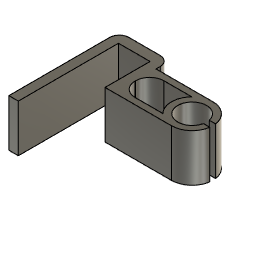
auto-top-off-clip (Autodesk Fusion 360 design; units mm, degrees)
Autodesk Fusion 360 part; units mm, degrees
note: some values were not read from the file. Set by a fixed rule: which sketch regions a step uses.
sketch "Sketch1" plane through (0, 0, 0) normal (0, 0, 1) x (1, 0, 0)
  line L0 (0, 0) -> (0, 31.75)
  line L1 (0, 31.75) -> (10, 31.75)
  line L2 (10, 31.75) -> (10, 15.875)
  line L3 (10, 15.875) -> (12, 15.875)
  line L4 (0, 0) -> (-3, 0)
  line L5 (-3, 0) -> (-3, 35)
  line L6 (-3, 35) -> (13, 35)
  line L7 (13, 35) -> (13, 17.5)
  line L8 (13, 17.5) -> (10, 17.5)
  circle A0 centre (31.0292, 24.0805) radius 4.572
  circle A1 centre (31.0292, 24.0805) radius 6.572
  line L9 (13, 17.5) -> (31.0468, 17.5)
  line L10 (31.0468, 17.5) -> (31.0468, 19.5)
  line L11 (31.0468, 19.5) -> (13, 19.5)
  line L12 (13, 19.5) -> (13, 17.5)
  line L13 (31.0292, 28.6525) -> (12.2404, 28.6525)
  line L14 (12.2404, 28.6525) -> (12.2404, 30.6525)
  line L15 (12.2404, 30.6525) -> (31.0292, 30.6525)
  line L16 (31.0292, 30.6525) -> (31.0292, 28.6525)
  line L17 (38, 25) -> (24.0584, 25)
  line L18 (24.0584, 25) -> (24.0584, 23.1611)
  line L19 (24.0584, 23.1611) -> (38, 23.1611)
  line L20 (38, 23.1611) -> (38, 25)
  line L21 (38, 25) -> (24.0584, 23.1611) construction
  line L22 (24.0584, 25) -> (38, 23.1611) construction
  point P0 (31.0292, 24.0805)
  dimension "d1" = 31.75
  dimension "d2" = 10
  dimension "d3" = 15.875
  dimension "d4" = 2
  dimension "d5" = 9.144
  dimension "d6" = 2
  dimension "d11" = 2
  dimension "d12" = 2
  constraint coincident L0.start L4.start
  constraint vertical L0
  constraint perpendicular L0 L1
  constraint perpendicular L1 L2
  constraint perpendicular L2 L3
  constraint perpendicular L0 L4
  constraint perpendicular L4 L5
  constraint perpendicular L5 L6
  constraint perpendicular L4 L7
  constraint coincident L2 L8.end
  constraint perpendicular L2 L8
  constraint horizontal L9
  constraint vertical L10
  constraint horizontal L11
  constraint vertical L12
  constraint horizontal L13
  constraint vertical L14
  constraint horizontal L15
  constraint vertical L16
  constraint coincident A0 L13.start
  constraint horizontal L17
  constraint perpendicular L17 L18
  constraint parallel L17 L19
  constraint parallel L18 L20
  constraint coincident L21 P0
  constraint coincident L22 P0
  constraint coincident P0 A0.centre
  measures "d1" distance of L0.start L0.end
  measures "d2" distance of L0.end L1.end
  measures "d3" distance of L1.end L2.end
  measures "d4" distance of L2.end L3.end
  measures "d5" diameter of A0
  measures "d11" distance of L7.end L11.end
  measures "d12" distance of L13.start L15.end
extrude "Extrude3" add sketch "Sketch1" along normal blind 15 contours L0 L1 L2 L4 L5 L6 L7 L8 L12 L13 L14 L15 | L7 A1 L9 L10 L11 L12 | L7 A1 L13 L15 | L7 L13 L14 L15 | A1 L13 L16 | A0 A1 L16 L17 | A1 L10 L11 | A0 A1 L10 L11 L19 | A0 A1 L13 L17 | A0 A1 L17 L19 picked at (25.8467, 24.7963)
sketch "Sketch3" plane through (0, 0, 10) normal (0, 0, 1) x (-1, 0, 0)
  line L0 (-13, -17.5) -> (-13, -35)
  line L1 (-13, -35) -> (3, -35)
  line L2 (3, -35) -> (3, 0)
  line L3 (3, 0) -> (0, 0)
  line L4 (0, 0) -> (0, -31.75)
  line L5 (0, -31.75) -> (-10, -31.75)
  line L6 (-10, -31.75) -> (-10, -17.5)
  line L7 (-10, -17.5) -> (-13, -17.5)
  circle A0 centre (-17.7478, -24.1114) radius 4.572
sketch "Sketch4" plane through (0, 0, 10) normal (0, 0, 1) x (-1, 0, 0)
  line L0 (-13, -17.5) -> (-13, -35)
  line L1 (-13, -35) -> (3, -35)
  line L2 (3, -35) -> (3, 0)
  line L3 (3, 0) -> (0, 0)
  line L4 (0, 0) -> (0, -31.75)
  line L5 (0, -31.75) -> (-10, -31.75)
  line L6 (-10, -31.75) -> (-10, -17.5)
  line L7 (-10, -17.5) -> (-13, -17.5)
  circle A0 centre (-17.7478, -24.1114) radius 4.572
  circle A1 centre (-17.7478, -24.1114) radius 6.572
  line L8 (-17.5, -22.5) -> (-17.5, -16.7493)
  constraint vertical L8
fillet "Fillet1" radius 4.5 2 edges at (13, 19.5, 7.5) (13, 28.6525, 7.5)
fillet "Fillet2" radius 3 2 edges at (13, 35, 7.5) (-3, 35, 7.5)
